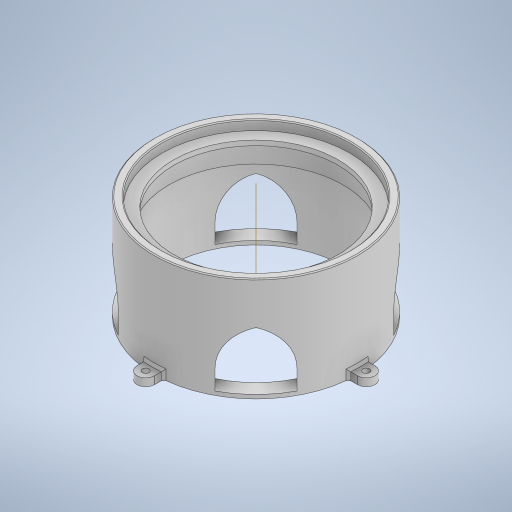
# Autodesk Inventor part: Base_BaseCircular
Saved by Autodesk Inventor 2023 (Build 270158000, 158)
## iProperties
Created: 2025-02-06
Part Number: Base_BaseCircular
Material: Generic
Document SubType Name: Modeling
Designer: Swoby
Density: 1 g/cm^3
Appearance: Default
Author: Swoby
Autodesk Inventor part; units mm, degrees
ref_plane "YZ Plane" through (0, 0, 0) normal (1, 0, 0) x (0, 1, 0)
ref_plane "XZ Plane" through (0, 0, 0) normal (0, 1, 0) x (-1, 0, 0)
sketch "Sketch1" plane through (0, 0, 0) normal (0, 0, 1) x (1, 0, 0)
  line L0 (0, 0) -> (0, 28.3025)
  line L1 (-52.5, 0) -> (-52.5, 53.7)
  line L2 (-52.5, 53.7) -> (-48.5, 53.7)
  line L3 (-48.5, 53.7) -> (-48.5, 48.7)
  line L4 (-48.5, 48.7) -> (-42.5, 48.7)
  line L5 (-42.5, 48.7) -> (-42.5, 46.2)
  line L6 (-42.5, 46.2) -> (-45, 36.2)
  line L7 (-45, 36.2) -> (-45, 0)
  line L8 (-52.5, 0) -> (-45, 0)
  dimension "d0" = 90
  dimension "d1" = 105
  dimension "d2" = 5
  dimension "d3" = 4
  dimension "d4" = 10
  dimension "d5" = 2.5
  dimension "d6" = 10
  dimension "d7" = 48.7
  constraints: 18 end point, 4 perpendicular, 2 vertical, 1 horizontal, 1 parallel, 1 point on line
  measures "d0" diameter of L7 L0
  measures "d1" diameter of L1 L0
  measures "d2" distance of L2.end L3.end
  measures "d3" distance of L1.end L2.end
  measures "d4" distance between parallel lines of L1 L5
  measures "d5" distance of L4.end L5.end
  measures "d6" vertical distance of L5.end L6.end
  measures "d7" distance between parallel lines of L8 L4
revolve "Revolution1" add sketch "Sketch1" angle 360 about axis through (0, 0, 0) along (0, 1, 0)
chamfer "Chamfer1" distance 0.5 angle 45 2 edges at (52.5, 53.7, 0) (48.5, 53.7, 0)
sketch "Sketch2" plane through (0, 0, 0) normal (0, -1, 0) x (1, 0, 0)
  line L0 (0, 0) -> (-57, 0) construction
  circle A0 centre (-57, 0) radius 1.75
  arc A1 (-52.5, 0) -> (-57, 4.5) centre (-57, 0) ccw construction
  circle A2 centre (0, 0) radius 52.5 projected
  line L1 (-57, -4.5) -> (-52.3068, -4.5)
  line L2 (-57, 4.5) -> (-52.3068, 4.5)
  arc A3 (-57, -4.5) -> (-52.5, 0) centre (-57, 0) ccw construction
  arc A4 (-57, 4.5) -> (-57, -4.5) centre (-57, 0) ccw
  dimension "d12" = 57
  dimension "d13" = 3.5
  dimension "d14" = 9
  constraints: 9 point on circle, 6 end point, 4 centre point, 4 tangent, 2 coincident, 2 horizontal, 1 parallel
  measures "d12" distance of L0.start L0.end
  measures "d13" diameter of A0
  measures "d14" diameter of A1
extrude "Extrusion1" add sketch "Sketch2" against normal blind 4 contours A2 L1 A4 L2
chamfer "Chamfer2" distance 1.2 angle 45 4 edges at (-52.4517, 4, -2.2521) (-52.4517, 4, 2.2521) (-52.3068, 2, 4.5) (-52.3068, 2, -4.5)
ref_plane "Work Plane1" through (0, 0, 0) normal (0.7071068, 0, -0.7071068) x (0, 1, 0)
sketch "Sketch3" plane through (0, 0, 0) normal (0.7071068, 0, -0.7071068) x (0, 1, 0)
  line L0 (36.2, -45) -> (36.2, 45) projected
  line L1 (0, -52.5) -> (0, 52.5) projected
  line L2 (36.2, -45) -> (36.2, 45) projected
  line L3 (0, -45) -> (0, 45) projected
  line L4 (0, 0) -> (36.2, 0)
  line L5 (2, 0) -> (2, -15)
  line L6 (2, -15) -> (12, -15)
  line L7 (12, -15) -> (12, 0)
  line L8 (12, 0) -> (32, 0)
  arc A0 (12, -15) -> (32, 0) centre (12, 5.8333) ccw
  line L9 (12, 0) -> (2, 0)
  line L10 (2, 0) -> (2, 15)
  line L11 (2, 15) -> (12, 15)
  line L12 (12, 15) -> (12, 0)
  arc A1 (32, 0) -> (12, 15) centre (12, -5.8333) ccw
  point P0 (0, -32.8776)
  point P1 (0, -40.9306)
  dimension "d21" = 2
  dimension "d22" = 10
  dimension "d23" = 30
  dimension "d24" = 20
  constraints: 18 end point, 4 point on circle, 3 point on line, 3 symmetric about line, 2 centre point, 2 perpendicular, 1 collinear, 1 midpoint, 1 tangent, 1 vertical, 1 other
  measures "d21" distance between parallel lines of L1 L5
  measures "d22" distance of L5.end L6.end
  measures "d23" diameter of L6 L4
  measures "d24" distance of L8.end L7.end
extrude "Extrusion2" cut sketch "Sketch3" against normal through all
pattern_circular "Circular Pattern1" count 4 over 360 about axis through (0, -10, 0) along (0, 1, 0) of "Extrusion2", "Extrusion1", "Chamfer2"
body "Solid1"
